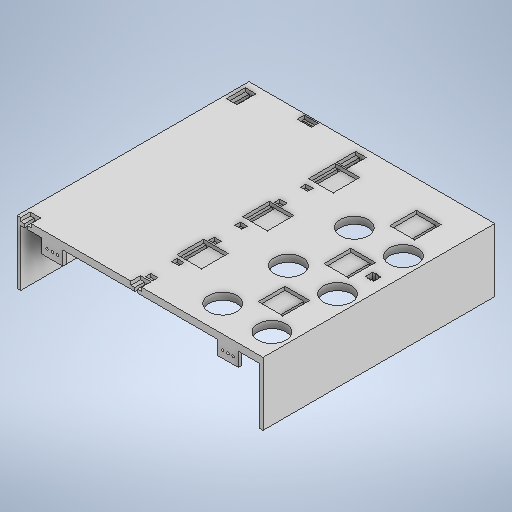
# Autodesk Inventor part: Højre
Saved by Autodesk Inventor 2025.2 (Build 292293000, 293)
## iProperties
Created: 2025-05-06
Part Number: Højre
Material: Generic
Document SubType Name: Modeling
Designer: lauri
Density: 1 g/cm^3
Appearance: Default
Author: lauri
Autodesk Inventor part; units mm, degrees
ref_plane "YZ Plane" through (0, 0, 0) normal (1, 0, 0) x (0, 1, 0)
ref_plane "XZ Plane" through (0, 0, 0) normal (0, 1, 0) x (-1, 0, 0)
ref_plane "XY Plane" through (0, 0, 0) normal (0, 0, 1) x (1, 0, 0)
sketch "Sketch1" plane through (0, 0, 0) normal (0, 1, 0) x (-1, 0, 0)
  line L0 (-175, 150) -> (175, 150)
  line L1 (175, 150) -> (175, -150)
  line L2 (175, -150) -> (-175, -150)
  line L3 (-175, -150) -> (-175, 150)
  line L4 (-175, 150) -> (175, -150) construction
  line L5 (175, 150) -> (-175, -150) construction
  point P0 (0, 0)
  point P1 (0, -180)
  point P2 (175, -180)
  dimension "d0" = 350
  dimension "d1" = 300
  constraints: 12 end point, 2 midpoint, 2 parallel, 1 horizontal, 1 perpendicular
  measures "d0" distance of L1.end L2.end
  measures "d1" distance of L0.end L1.end
extrude "Extrusion1" add sketch "Sketch1" along normal blind 10
sketch "Sketch2" plane through (0, 10, 0) normal (0, 1, 0) x (1, 0, 0)
  line L0 (-175, 150) -> (-175, -150) projected
  line L1 (-175, -150) -> (-170, -150)
  line L2 (-170, -150) -> (-155, -150)
  line L3 (-155, -150) -> (-155, -136.5)
  line L4 (-155, -136.5) -> (-170, -136.5)
  line L5 (-170, -136.5) -> (-170, -150)
  line L6 (-175, -150) -> (175, -150) projected
  line L7 (-13, -150) -> (2, -150)
  line L8 (2, -150) -> (2, -136.5)
  line L9 (2, -136.5) -> (-13, -136.5)
  line L10 (-13, -136.5) -> (-13, -150)
  line L11 (175, 150) -> (-175, 150) projected
  point P0 (0, 0)
  point P1 (-13, 108)
  point P2 (-170, 108)
  dimension "d4" = 5
  dimension "d5" = 15
  dimension "d6" = 13.5
  dimension "d8" = 15
  dimension "d9" = 13.5
  constraints: 18 end point, 4 parallel, 3 horizontal, 2 perpendicular, 1 point on line
  measures "d4" distance of L0.end L1.end
  measures "d5" distance of L4.end L3.end
  measures "d6" distance of L3.end L2.end
  measures "d8" distance of L9.end L8.end
  measures "d9" distance of L8.end L7.end
extrude "Extrusion2" cut sketch "Sketch2" against normal blind 5
sketch "Sketch3" plane through (0, 10, 0) normal (0, 1, 0) x (1, 0, 0)
  line L0 (2, -136.5) -> (2, -150) projected
  line L1 (-13, -150) -> (-13, -136.5) projected
  line L2 (-7.5, -150) -> (-3.5, -150)
  line L3 (-3.5, -150) -> (-3.5, -136.5)
  line L4 (-3.5, -136.5) -> (-7.5, -136.5)
  line L5 (-7.5, -136.5) -> (-7.5, -150)
  line L6 (-7.5, -150) -> (-3.5, -136.5) construction
  line L7 (-3.5, -150) -> (-7.5, -136.5) construction
  line L8 (-155, -136.5) -> (-155, -150) projected
  line L9 (-170, -150) -> (-170, -136.5) projected
  line L10 (-164.5, -150) -> (-160.5, -150)
  line L11 (-160.5, -150) -> (-160.5, -136.5)
  line L12 (-160.5, -136.5) -> (-164.5, -136.5)
  line L13 (-164.5, -136.5) -> (-164.5, -150)
  line L14 (-164.5, -150) -> (-160.5, -136.5) construction
  line L15 (-160.5, -150) -> (-164.5, -136.5) construction
  point P0 (0, 0)
  point P1 (-5.5, -143.25)
  point P2 (-162.5, -143.25)
  dimension "d15" = 4
  dimension "d16" = 13.5
  dimension "d17" = 4
  dimension "d18" = 13.5
  constraints: 24 end point, 4 midpoint, 4 parallel, 2 horizontal, 2 perpendicular
  measures "d15" distance of L4.end L3.end
  measures "d16" distance of L3.end L2.end
  measures "d17" distance of L12.end L11.end
  measures "d18" distance of L11.end L10.end
extrude "Extrusion3" cut sketch "Sketch3" against normal through all
sketch "Sketch11" plane through (0, 0, 0) normal (0, -1, 0) x (1, 0, 0)
  line L0 (170, 150) -> (170, -145) projected
  line L1 (170, 150) -> (140, 150)
  line L2 (140, 150) -> (140, 145)
  line L3 (170, 145) -> (170, 150)
  line L4 (-170, 150) -> (-170, -145) projected
  line L5 (-140, 150) -> (-110, 150)
  line L6 (-110, 150) -> (-110, 145)
  line L7 (-110, 145) -> (-140, 145)
  line L8 (-140, 145) -> (-140, 150)
  line L9 (140, 150) -> (110, 150)
  line L10 (110, 150) -> (110, 145)
  line L11 (110, 145) -> (140, 145)
  line L12 (140, 145) -> (140, 150)
  point P0 (0, 0)
  dimension "d96" = 30
  dimension "d97" = 5
  dimension "d98" = 30
  dimension "d99" = 30
  dimension "d100" = 5
  dimension "d101" = 30
  dimension "d102" = 5
  constraints: 22 end point, 5 parallel, 3 horizontal, 3 perpendicular
  measures "d96" distance of L3.start L2.end
  measures "d97" distance of L2.end L1.end
  measures "d98" distance of L4.start L5.start
  measures "d99" distance of L6.end L7.end
  measures "d100" distance of L5.end L6.end
  measures "d101" distance of L11.end L10.end
  measures "d102" distance of L10.end L9.end
extrude "Extrusion9" add sketch "Sketch11" along normal blind 20
sketch "Sketch12" plane through (-155, 10, 150) normal (0, 0, 1) x (1, 0, 0)
  line L0 (295, -10) -> (295, -30) projected
  line L1 (295, -20) -> (265, -20)
  line L2 (265, -10) -> (265, -30) projected
  line L3 (45, -10) -> (45, -30) projected
  line L4 (45, -20) -> (15, -20)
  line L5 (15, -10) -> (15, -30) projected
  point P0 (155, -10)
  point P1 (280, -20)
  point P2 (287.5, -20)
  point P3 (272.5, -20)
  point P4 (30, -20)
  point P5 (37.5, -20)
  point P6 (22.5, -20)
  constraints: 6 midpoint, 4 end point, 4 point on line
hole "Hole2" at (125, -10, 150) at (132.5, -10, 150) at (117.5, -10, 150) at (-125, -10, 150) at (-117.5, -10, 150) at (-132.5, -10, 150) direction (0, 0, -1) diameter 3.5 depth 5
sketch "Sketch14" plane through (175, 10, -150) normal (0, 0, -1) x (-1, 0, 0)
  line L0 (350, -90) -> (0, -90) projected
  line L1 (0, -90) -> (50, -90)
  line L2 (50, -90) -> (50, -70)
  line L3 (350, -90) -> (300, -90)
  line L4 (300, -90) -> (300, -70)
  point P0 (175, -10)
  point P1 (57.5, -40)
  point P2 (42.5, -40)
  point P3 (307.5, -40)
  point P4 (292.5, -40)
  dimension "d122" = 50
  dimension "d123" = 20
  dimension "d124" = 50
  dimension "d125" = 20
  constraints: 8 end point, 2 coincident, 2 perpendicular, 2 point on line
  measures "d122" distance of L0.end L1.end
  measures "d123" distance of L1.end L2.end
  measures "d124" distance of L0.start L3.end
  measures "d125" distance of L3.end L4.end
hole "Hole3" at (125, -60, -150) at (117.5, -30, -150) at (132.5, -30, -150) at (-125, -60, -150) at (-132.5, -30, -150) at (-117.5, -30, -150) direction (0, 0, 1) diameter 3.5 depth 5
sketch "Sketch17" plane through (0, 10, 0) normal (0, 1, 0) x (1, 0, 0)
  line L0 (2, -136.5) -> (2, -134)
  line L1 (2, -134) -> (-8.1, -134)
  line L2 (-8.1, -134) -> (-8.1, -126.4)
  line L3 (-8.1, -126.4) -> (2, -126.4)
  line L4 (2, -126.4) -> (2, -134)
  line L5 (2, -130.2) -> (2, -96.95)
  line L6 (2, -96.95) -> (-8.1, -96.95)
  line L7 (-8.1, -96.95) -> (-8.1, -89.35)
  line L8 (-8.1, -89.35) -> (2, -89.35)
  line L9 (2, -89.35) -> (2, -96.95)
  line L10 (-13, -150) -> (-13, -136.5) projected
  line L11 (-13, -84.6) -> (22.1, -84.6)
  line L12 (22.1, -84.6) -> (22.1, -46.7)
  line L13 (22.1, -46.7) -> (-13, -46.7)
  line L14 (-13, -46.7) -> (-13, -84.6)
  line L15 (2, -44.05) -> (-8.1, -44.05)
  line L16 (-8.1, -44.05) -> (-8.1, -36.45)
  line L17 (-8.1, -36.45) -> (2, -36.45)
  line L18 (2, -36.45) -> (2, -44.05)
  line L19 (2, -36.45) -> (2, -6.95)
  line L20 (2, -6.95) -> (-8.1, -6.95)
  line L21 (-8.1, -6.95) -> (-8.1, 0.65)
  line L22 (-8.1, 0.65) -> (2, 0.65)
  line L23 (2, 0.65) -> (2, -6.95)
  line L24 (-13, -46.7) -> (-13, 9.05)
  line L25 (-13, 9.05) -> (22.1, 9.05)
  line L26 (22.1, 9.05) -> (22.1, 46.95)
  line L27 (22.1, 46.95) -> (-13, 46.95)
  line L28 (-13, 46.95) -> (-13, 9.05)
  line L29 (2, 49.5) -> (-8.1, 49.5)
  line L30 (-8.1, 49.5) -> (-8.1, 57.1)
  line L31 (-8.1, 57.1) -> (2, 57.1)
  line L32 (2, 57.1) -> (2, 49.5)
  line L33 (2, 57.1) -> (2, 86.6)
  line L34 (2, 86.6) -> (-8.1, 86.6)
  line L35 (-8.1, 86.6) -> (-8.1, 94.2)
  line L36 (-8.1, 94.2) -> (2, 94.2)
  line L37 (2, 94.2) -> (2, 86.6)
  line L38 (-13, 46.95) -> (-13, 102.7)
  line L39 (-13, 102.7) -> (22.1, 102.7)
  line L40 (22.1, 102.7) -> (22.1, 140.6)
  line L41 (22.1, 140.6) -> (-13, 140.6)
  line L42 (-13, 140.6) -> (-13, 102.7)
  line L43 (-13, 142.9) -> (-13, 169.9)
  line L44 (-13, 169.9) -> (2, 169.9)
  line L45 (2, 169.9) -> (2, 142.9)
  line L46 (2, 142.9) -> (-13, 142.9)
  line L47 (2, 142.9) -> (-170, 142.9)
  line L48 (-175, 150) -> (-175, -150) projected
  line L49 (-170, 142.9) -> (-155, 142.9)
  line L50 (-155, 142.9) -> (-155, 169.9)
  line L51 (-155, 169.9) -> (-170, 169.9)
  line L52 (-170, 169.9) -> (-170, 142.9)
  line L53 (-13, -46.7) -> (138, -46.7)
  line L54 (-13, 46.95) -> (138, 46.95)
  line L55 (-13, 140.6) -> (138, 140.6)
  line L56 (138, 140.6) -> (102.9, 140.6)
  line L57 (102.9, 140.6) -> (102.9, 102.7)
  line L58 (102.9, 102.7) -> (138, 102.7)
  line L59 (138, 102.7) -> (138, 140.6)
  line L60 (138, 46.95) -> (102.9, 46.95)
  line L61 (102.9, 46.95) -> (102.9, 9.05)
  line L62 (102.9, 9.05) -> (138, 9.05)
  line L63 (138, 9.05) -> (138, 46.95)
  line L64 (138, -46.7) -> (102.9, -46.7)
  line L65 (102.9, -46.7) -> (102.9, -84.6)
  line L66 (102.9, -84.6) -> (138, -84.6)
  line L67 (138, -84.6) -> (138, -46.7)
  line L68 (2, 0.65) -> (2, 51.1052)
  point P0 (0, 0)
  point P1 (102.9, -46.7)
  point P2 (102.9, 46.95)
  point P3 (102.9, 140.6)
  dimension "d141" = 2.5
  dimension "d142" = 10.1
  dimension "d143" = 7.6
  dimension "d144" = 33.25
  dimension "d145" = 7.6
  dimension "d147" = 35.1
  dimension "d148" = 37.9
  dimension "d149" = 45.3
  dimension "d150" = 10.1
  dimension "d151" = 7.6
  dimension "d152" = 29.5
  dimension "d153" = 7.6
  dimension "d154" = 55.75
  dimension "d155" = 37.9
  dimension "d157" = 7.6
  dimension "d158" = 29.5
  dimension "d159" = 7.6
  dimension "d160" = 55.75
  dimension "d161" = 37.9
  dimension "d166" = 27
  dimension "d167" = 15
  dimension "d168" = 172
  dimension "d169" = 15
  dimension "d170" = 27
  dimension "d203" = 151
  dimension "d204" = 151
  dimension "d205" = 151
  dimension "d206" = 35.1
  dimension "d273" = 35.1
  dimension "d274" = 35.1
  dimension "d275" = 37.9
  dimension "d276" = 37.9
  dimension "d277" = 37.9
  dimension "d278" = 35.1
  dimension "d279" = 35.1
  dimension "d280" = 10.1
  dimension "d281" = 10.1
  dimension "d282" = 10.1
  dimension "d283" = 10.1
  constraints: 134 end point, 26 parallel, 17 perpendicular, 15 horizontal, 8 vertical, 3 point on line, 1 coincident, 1 midpoint
  measures "d141" distance of L0.start L0.end
  measures "d142" distance of L2.end L3.end
  measures "d143" distance of L1.end L2.end
  measures "d144" distance of L5.start L5.end
  measures "d145" distance of L6.end L7.end
  measures "d147" distance of L13.end L12.end
  measures "d148" distance of L12.end L11.end
  measures "d149" distance of L8.end L15.start
  measures "d150" distance of L16.end L17.end
  measures "d151" distance of L15.end L16.end
  measures "d152" distance of L17.end L19.end
  measures "d153" distance of L20.end L21.end
  measures "d154" distance of L13.end L24.end
  measures "d155" distance of L26.end L25.end
  measures "d157" distance of L29.end L30.end
  measures "d158" distance of L31.end L33.end
  measures "d159" distance of L34.end L35.end
  measures "d160" distance of L27.end L38.end
  measures "d161" distance of L40.end L39.end
  measures "d166" distance of L43.start L43.end
  measures "d167" distance of L43.end L44.end
  measures "d168" distance of L45.end L47.end
  measures "d169" distance of L51.end L50.end
  measures "d170" distance of L50.end L49.end
  measures "d203" distance of L13.end L53.end
  measures "d204" distance of L27.end L54.end
  measures "d205" distance of L41.end L55.end
  measures "d206" distance of L58.end L57.end
  measures "d273" distance of L24.end L25.end
  measures "d274" distance of L38.end L39.end
  measures "d275" distance of L56.end L57.end
  measures "d276" distance of L60.end L61.end
  measures "d277" distance of L66.end L53.end
  measures "d278" distance of L65.end L66.end
  measures "d279" distance of L61.end L62.end
  measures "d280" distance of L7.end L8.end
  measures "d281" distance of L21.end L22.end
  measures "d282" distance of L30.end L31.end
  measures "d283" distance of L33.end L34.end
sketch "Sketch19" plane through (0, 10, 0) normal (0, 1, 0) x (1, 0, 0)
  line L0 (-175, 150) -> (175, 150) projected
  line L1 (-175, 150) -> (175, 150)
  line L2 (175, 150) -> (175, 180)
  line L3 (175, 180) -> (-175, 180)
  line L4 (-175, 180) -> (-175, 150)
  point P0 (0, 0)
  dimension "d163" = 30
  constraints: 8 end point, 2 parallel, 1 horizontal, 1 perpendicular
  measures "d163" distance of L2.end L1.end
extrude "Extrusion13" add sketch "Sketch19" against normal blind 10
sketch "Sketch20" plane through (0, 0, 0) normal (0, -1, 0) x (1, 0, 0)
  line L0 (-175, 150) -> (-175, -180) projected
  line L1 (175, 150) -> (175, -180) projected
  line L2 (-175, -180) -> (175, -180)
  line L3 (175, -180) -> (175, -175)
  line L4 (175, -175) -> (-175, -175)
  line L5 (-175, -175) -> (-175, -180)
  line L6 (175, -180) -> (170, -180)
  line L7 (170, -180) -> (170, 150)
  line L8 (170, 150) -> (175, 150)
  line L9 (175, 150) -> (175, -180)
  line L10 (-170, 150) -> (-170, 136.5) projected
  line L11 (-175, -180) -> (-170, -180)
  line L12 (-170, -180) -> (-170, 150)
  line L13 (-170, 150) -> (-175, 150)
  line L14 (-175, 150) -> (-175, -180)
  point P0 (0, 0)
  point P1 (170, -175)
  point P2 (-170, -175)
  point P3 (175, -180)
  dimension "d174" = 5
  dimension "d175" = 5
  dimension "d176" = 5
  constraints: 24 end point, 6 parallel, 3 horizontal, 3 perpendicular, 1 point on line
  measures "d174" distance of L3.end L2.end
  measures "d175" distance of L7.end L8.end
  measures "d176" distance of L13.end L10.start
extrude "Extrusion15" add sketch "Sketch20" along normal blind 80
sketch "Sketch21" plane through (175, 10, -180) normal (0, 0, -1) x (-1, 0, 0)
  line L0 (350, -90) -> (350, 0) projected
  line L1 (350, 0) -> (300, 0)
  line L2 (0, 0) -> (350, 0) projected
  line L3 (300, 0) -> (300, -70)
  line L4 (0, 0) -> (50, 0)
  line L5 (50, 0) -> (50, -70)
  point P0 (175, -10)
  point P1 (307.5, -40)
  point P2 (292.5, -40)
  point P3 (57.5, -40)
  point P4 (42.5, -40)
  dimension "d179" = 50
  dimension "d180" = 70
  dimension "d181" = 50
  dimension "d182" = 70
  constraints: 8 end point, 2 coincident, 2 perpendicular, 2 point on line
  measures "d179" distance of L0.end L1.end
  measures "d180" distance of L1.end L3.end
  measures "d181" distance of L2.start L4.end
  measures "d182" distance of L4.end L5.end
hole "Hole4" at (-132.5, -30, -180) at (-117.5, -30, -180) at (-125, -60, -180) at (117.5, -30, -180) at (125, -60, -180) at (132.5, -30, -180) direction (0, 0, 1) diameter 3.5 end through all
sketch "Sketch22" plane through (0, 10, 0) normal (0, 1, 0) x (1, 0, 0)
  line L0 (-170, 169.9) -> (-155, 169.9) projected
  line L1 (-155, 169.9) -> (-13.4835, 169.9)
  line L2 (-84.2417, 169.9) -> (-84.2417, 178)
  line L3 (-84.2417, 178) -> (-94.2417, 178)
  line L4 (-94.2417, 178) -> (-74.2417, 178)
  line L5 (-74.2417, 178) -> (-74.2417, 168)
  line L6 (-74.2417, 168) -> (-94.2417, 168)
  line L7 (-94.2417, 168) -> (-94.2417, 178)
  point P0 (0, 0)
  dimension "d190" = 8.1
  dimension "d191" = 10
  dimension "d192" = 20
  dimension "d193" = 10
  constraints: 14 end point, 3 horizontal, 2 parallel, 1 midpoint, 1 perpendicular, 1 vertical
  measures "d190" distance of L2.start L2.end
  measures "d191" distance of L2.end L3.end
  measures "d192" distance of L5.end L6.end
  measures "d193" distance of L4.end L5.end
extrude "Extrusion16" cut sketch "Sketch22" against normal blind 5
sketch "Sketch23" plane through (-175, 10, -180) normal (-1, 0, 0) x (0, 0, 1)
  line L0 (170.95, -5) -> (170.95, -10)
  line L1 (133.15, -10) -> (133.15, -5)
  line L2 (264.5, -5) -> (264.5, -10)
  line L3 (226.7, -10) -> (226.7, -5)
  line L4 (39.6, -5) -> (77.4, -5)
  line L5 (77.4, -5) -> (77.4, -10)
  line L6 (39.6, -10) -> (39.6, -5)
  line L7 (255.6, -2.5) -> (235.6, -2.5)
  line L8 (235.6, -2.5) -> (235.6, -7.5)
  line L9 (235.6, -7.5) -> (255.6, -7.5)
  line L10 (255.6, -7.5) -> (255.6, -2.5)
  line L11 (255.6, -2.5) -> (235.6, -7.5) construction
  line L12 (235.6, -2.5) -> (255.6, -7.5) construction
  line L13 (162.05, -7.5) -> (142.05, -7.5)
  line L14 (142.05, -7.5) -> (142.05, -2.5)
  line L15 (142.05, -2.5) -> (162.05, -2.5)
  line L16 (162.05, -2.5) -> (162.05, -7.5)
  line L17 (162.05, -7.5) -> (142.05, -2.5) construction
  line L18 (142.05, -7.5) -> (162.05, -2.5) construction
  line L19 (68.5, -7.5) -> (48.5, -7.5)
  line L20 (48.5, -7.5) -> (48.5, -2.5)
  line L21 (48.5, -2.5) -> (68.5, -2.5)
  line L22 (68.5, -2.5) -> (68.5, -7.5)
  line L23 (68.5, -7.5) -> (48.5, -2.5) construction
  line L24 (48.5, -7.5) -> (68.5, -2.5) construction
  point P0 (180, -10)
  point P1 (245.6, -5)
  point P2 (152.05, -5)
  point P3 (58.5, -5)
  dimension "d196" = 5
  dimension "d197" = 5
  dimension "d198" = 5
  dimension "d292" = 20
  dimension "d293" = 20
  dimension "d294" = 20
  constraints: 50 end point, 9 parallel, 6 midpoint, 4 horizontal, 4 perpendicular
  measures "d196" distance of L0.start L0.end
  measures "d197" distance of L2.start L2.end
  measures "d198" distance of L4.end L5.end
  measures "d292" distance of L9.end L8.end
  measures "d293" distance of L14.end L15.end
  measures "d294" distance of L20.end L21.end
extrude "Extrusion18" cut sketch "Sketch17" against normal blind 5
sketch "Sketch24" plane through (0, 10, 0) normal (0, 1, 0) x (1, 0, 0)
  line L0 (102.9, -46.7) -> (138, -46.7) projected
  line L1 (138, 9.05) -> (138, -46.7)
  line L2 (138, -18.825) -> (175, -18.825)
  line L3 (175, -150) -> (175, 180) projected
  line L4 (138, 46.95) -> (138, 9.05) projected
  line L5 (138, 102.7) -> (102.9, 102.7) projected
  line L6 (138, 46.95) -> (138, 102.7)
  line L7 (138, 74.825) -> (175, 74.825)
  line L8 (22.1, 46.95) -> (22.1, 9.05) projected
  line L9 (22.1, -46.7) -> (22.1, -84.6) projected
  line L10 (22.1, 9.05) -> (22.1, -46.7)
  line L11 (22.1, 46.95) -> (22.1, 102.7)
  line L12 (138, -18.825) -> (22.1, -18.825)
  line L13 (22.1, 74.825) -> (138, 74.825)
  line L14 (150, -18.825) -> (150, -112.375)
  point P0 (0, 0)
  point P1 (80.05, -18.825)
  point P2 (80.05, 74.825)
  point P3 (150, 74.825)
  point P4 (80, -112.375)
  dimension "d251" = 93.55
  constraints: 18 end point, 6 midpoint, 5 vertical, 4 point on line, 1 coincident, 1 horizontal, 1 parallel, 1 perpendicular
  measures "d251" distance of L14.start L14.end
sketch "Sketch25" plane through (0, 10, 0) normal (0, 1, 0) x (1, 0, 0)
  circle A0 centre (154, -18.825) radius 15 projected
  circle A1 centre (154, 74.725) radius 15 projected
  line L0 (154, -18.825) -> (154, 74.725)
  line L1 (160, 22.95) -> (148, 22.95)
  line L2 (148, 22.95) -> (148, 32.95)
  line L3 (148, 32.95) -> (160, 32.95)
  line L4 (160, 32.95) -> (160, 22.95)
  line L5 (160, 22.95) -> (148, 32.95) construction
  line L6 (148, 22.95) -> (160, 32.95) construction
  line L7 (154, 32.95) -> (154, 33.15)
  line L8 (154, 22.95) -> (154, 22.75)
  line L9 (156.15, 22.7397) -> (151.85, 22.7397)
  line L10 (151.85, 22.7397) -> (151.85, 22.2397)
  line L11 (151.85, 22.2397) -> (156.15, 22.2397)
  line L12 (156.15, 22.2397) -> (156.15, 22.7397)
  line L13 (156.15, 33.15) -> (151.85, 33.15)
  line L14 (151.85, 33.15) -> (151.85, 33.65)
  line L15 (151.85, 33.65) -> (156.15, 33.65)
  line L16 (156.15, 33.65) -> (156.15, 33.15)
  point P0 (0, 0)
  point P1 (154, 27.95)
  dimension "d223" = 12
  dimension "d224" = 10
  dimension "d225" = 0.2
  dimension "d226" = 0.2
  dimension "d227" = 0.5
  dimension "d228" = 0.5
  constraints: 34 end point, 6 parallel, 5 midpoint, 3 horizontal, 3 perpendicular, 2 point on line, 1 vertical
  measures "d223" distance of L2.end L3.end
  measures "d224" distance of L1.end L2.end
  measures "d225" distance of L7.start L7.end
  measures "d226" distance of L8.start L8.end
  measures "d227" distance of L10.end L9.end
  measures "d228" distance of L13.end L14.end
extrude "Extrusion19" cut sketch "Sketch25" against normal blind 10 contours L13 L14 L15 L0 | L0 L15 L16 L13 | L1 L2 L3 L0 | L0 L3 L4 L1 | L11 L10 L9 L0 | L0 L9 L12 L11
sketch "Sketch26" plane through (0, 10, 0) normal (0, 1, 0) x (1, 0, 0)
  line L0 (-155, 169.9) -> (-155, 142.9) projected
  line L1 (-155, 156.4) -> (-170, 156.4)
  line L2 (-170, 175) -> (-170, -150) projected
  line L3 (-170, 169.9) -> (-155, 169.9) projected
  line L4 (-164.5, 142.9) -> (-160.5, 142.9)
  line L5 (-160.5, 142.9) -> (-160.5, 169.9)
  line L6 (-160.5, 169.9) -> (-164.5, 169.9)
  line L7 (-164.5, 169.9) -> (-164.5, 142.9)
  line L8 (-164.5, 142.9) -> (-160.5, 169.9) construction
  line L9 (-160.5, 142.9) -> (-164.5, 169.9) construction
  line L10 (2, 169.9) -> (2, 142.9) projected
  line L11 (2, 156.4) -> (-13, 156.4)
  line L12 (-13, 142.9) -> (-13, 169.9) projected
  line L13 (-3.5, 142.9) -> (-7.5, 142.9)
  line L14 (-7.5, 142.9) -> (-7.5, 169.9)
  line L15 (-7.5, 169.9) -> (-3.5, 169.9)
  line L16 (-3.5, 169.9) -> (-3.5, 142.9)
  line L17 (-3.5, 142.9) -> (-7.5, 169.9) construction
  line L18 (-7.5, 142.9) -> (-3.5, 169.9) construction
  line L19 (-74.2417, 168) -> (-94.2417, 168) projected
  line L20 (-175, 180) -> (175, 180) projected
  line L21 (-94.2417, 168) -> (-94.2417, 178) projected
  line L22 (-74.2417, 171) -> (-94.2417, 171)
  line L23 (-94.2417, 171) -> (-94.2417, 175)
  line L24 (-94.2417, 175) -> (-74.2417, 175)
  line L25 (-74.2417, 175) -> (-74.2417, 171)
  line L26 (-74.2417, 171) -> (-94.2417, 175) construction
  line L27 (-94.2417, 171) -> (-74.2417, 175) construction
  line L28 (138, 140.6) -> (138, 102.7) projected
  line L29 (138, 121.65) -> (132, 121.65)
  line L30 (138, 46.95) -> (138, 9.05) projected
  line L31 (138, 28) -> (132, 28)
  line L32 (138, -46.7) -> (138, -84.6) projected
  line L33 (138, -65.65) -> (132, -65.65)
  line L34 (-13, -84.6) -> (-13, -46.7) projected
  line L35 (-13, -65.65) -> (-7, -65.65)
  line L36 (-13, 9.05) -> (-13, 46.95) projected
  line L37 (-13, 28) -> (-7, 28)
  line L38 (-13, 102.7) -> (-13, 140.6) projected
  line L39 (-13, 121.65) -> (-7, 121.65)
  line L40 (-13, -46.7) -> (22.1, -46.7) projected
  line L41 (-9, -84.6) -> (-5, -84.6)
  line L42 (-5, -84.6) -> (-5, -46.7)
  line L43 (-5, -46.7) -> (-9, -46.7)
  line L44 (-9, -46.7) -> (-9, -84.6)
  line L45 (-9, -84.6) -> (-5, -46.7) construction
  line L46 (-5, -84.6) -> (-9, -46.7) construction
  line L47 (-9, 9.1) -> (-5, 9.1)
  line L48 (-5, 9.1) -> (-5, 46.9)
  line L49 (-5, 46.9) -> (-9, 46.9)
  line L50 (-9, 46.9) -> (-9, 9.1)
  line L51 (-9, 9.1) -> (-5, 46.9) construction
  line L52 (-5, 9.1) -> (-9, 46.9) construction
  line L53 (-9, 140.55) -> (-5, 140.55)
  line L54 (-5, 140.55) -> (-5, 102.75)
  line L55 (-5, 102.75) -> (-9, 102.75)
  line L56 (-9, 102.75) -> (-9, 140.55)
  line L57 (-9, 140.55) -> (-5, 102.75) construction
  line L58 (-5, 140.55) -> (-9, 102.75) construction
  line L59 (102.9, -46.7) -> (138, -46.7) projected
  line L60 (134, -84.6) -> (130, -84.6)
  line L61 (130, -84.6) -> (130, -46.7)
  line L62 (130, -46.7) -> (134, -46.7)
  line L63 (134, -46.7) -> (134, -84.6)
  line L64 (134, -84.6) -> (130, -46.7) construction
  line L65 (130, -84.6) -> (134, -46.7) construction
  line L66 (134.004, 9.0994) -> (129.996, 9.0994)
  line L67 (129.996, 9.0994) -> (129.996, 46.9006)
  line L68 (129.996, 46.9006) -> (134.004, 46.9006)
  line L69 (134.004, 46.9006) -> (134.004, 9.0994)
  line L70 (134.004, 9.0994) -> (129.996, 46.9006) construction
  line L71 (129.996, 9.0994) -> (134.004, 46.9006) construction
  line L72 (102.9, 140.6) -> (138, 140.6) projected
  line L73 (134.004, 102.7) -> (129.996, 102.7)
  line L74 (129.996, 102.7) -> (129.996, 140.6)
  line L75 (129.996, 140.6) -> (134.004, 140.6)
  line L76 (134.004, 140.6) -> (134.004, 102.7)
  line L77 (134.004, 102.7) -> (129.996, 140.6) construction
  line L78 (129.996, 102.7) -> (134.004, 140.6) construction
  point P0 (0, 0)
  point P1 (-162.5, 156.4)
  point P2 (-5.5, 156.4)
  point P3 (-94.2417, 180)
  point P4 (-84.2417, 173)
  dimension "d231" = 4
  dimension "d232" = 4
  dimension "d233" = 4
  dimension "d234" = 6
  dimension "d235" = 6
  dimension "d236" = 6
  dimension "d237" = 6
  dimension "d238" = 6
  dimension "d239" = 4
  dimension "d240" = 4
  dimension "d241" = 4
  constraints: 124 end point, 29 midpoint, 18 parallel, 16 horizontal, 9 perpendicular, 7 point on line
  measures "d231" distance of L6.end L5.end
  measures "d232" distance of L14.end L15.end
  measures "d233" distance of L22.end L23.end
  measures "d234" distance of L29.start L29.end
  measures "d235" distance of L31.start L31.end
  measures "d236" distance of L33.start L33.end
  measures "d237" distance of L35.start L35.end
  measures "d238" distance of L37.start L37.end
  measures "d239" distance of L43.end L42.end
  measures "d240" distance of L49.end L48.end
  measures "d241" distance of L61.end L62.end
extrude "Extrusion20" cut sketch "Sketch26" against normal blind 10 contours L5 L1 L7 L3 | L5 L4 L7 L1 | L16 L13 L14 L11 | L11 L14 L15 L16 | L21 L24 L25 L22 | L76 L73 L74 L72 | L63 L60 L61 L59 | L44 L40 L42 L41 | L50 L49 L48 L47 | L53 L54 L55 L56 | L66 L67 L68 L69
sketch "Sketch27" plane through (175, 10, -180) normal (0, 0, -1) x (-1, 0, 0)
  line L0 (350, 0) -> (350, -90) projected
  line L1 (350, -45) -> (0, -45)
  line L2 (0, 0) -> (0, -90) projected
  point P0 (175, -10)
  point P1 (175, -45)
  constraints: 3 midpoint, 2 end point
hole "Hole9" at (0, -35, -180) direction (0, 0, 1) diameter 40 depth 30
hole "Hole10" at (80.05, 10, 18.825) at (80.05, 10, -74.825) at (150, 10, 18.825) at (150, 10, -74.825) at (150, 10, 112.375) at (80, 10, 112.375) direction (0, -1, 0) diameter 40 depth 30
sketch "Sketch28" plane through (0, 10, 0) normal (0, 1, 0) x (1, 0, 0)
  line L0 (2, -126.4) -> (2, -134) projected
  line L1 (2, -130.2) -> (-0.517, -130.2)
  line L2 (2, -89.35) -> (2, -96.95) projected
  line L3 (2, -93.15) -> (-0.517, -93.15)
  line L4 (2, -36.45) -> (2, -44.05) projected
  line L5 (2, -40.25) -> (-0.517, -40.25)
  line L6 (2, 0.65) -> (2, -6.95) projected
  line L7 (2, -3.15) -> (-0.517, -3.15)
  line L8 (2, 57.1) -> (2, 49.5) projected
  line L9 (2, 53.3) -> (-0.517, 53.3)
  line L10 (2, 94.2) -> (2, 86.6) projected
  line L11 (2, 90.4) -> (-0.517, 90.4)
  point P0 (0, 0)
  dimension "d284" = 2.517
  constraints: 12 end point, 6 coincident, 6 horizontal, 6 midpoint
  measures "d284" distance of L1.start L1.end
hole "Hole11" at (-0.517, 10, 130.2) at (-0.517, 10, 93.15) at (-0.517, 10, 40.25) at (-0.517, 10, 3.15) at (-0.517, 10, -53.3) at (-0.517, 10, -90.4) direction (0, -1, 0) diameter 3.5 depth 10
extrude "Extrusion21" cut sketch "Sketch23" against normal blind 10
body "Solid1"
